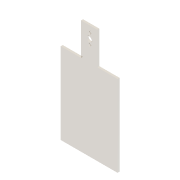
# Autodesk Inventor part: Ball Release
Saved by Autodesk Inventor 2015 SP1 (Build 190203100, 203)
## iProperties
Created: 2014-09-15
Part Number: Ball Release
Document SubType Name: Modeling
Designer: Family Room
Density: 1 g/cm^3
Material: Generic
Appearance: Polycarbonate - Smoked
Author: Family Room
Autodesk Inventor part; units mm, degrees
ref_plane "YZ Plane" through (0, 0, 0) normal (1, 0, 0) x (0, 1, 0)
ref_plane "XZ Plane" through (0, 0, 0) normal (0, 1, 0) x (-1, 0, 0)
ref_plane "XY Plane" through (0, 0, 0) normal (0, 0, 1) x (1, 0, 0)
sketch "Sketch1" plane through (0, 0, 0) normal (0, 0, 1) x (1, 0, 0)
  line L0 (0, 0) -> (88.9, 0)
  line L1 (88.9, 0) -> (88.9, 76.2)
  line L2 (0, 76.2) -> (0, 0)
  line L3 (57.15, 76.2) -> (57.15, 127)
  line L4 (57.15, 127) -> (31.75, 127)
  line L5 (31.75, 127) -> (31.75, 76.2)
  circle A0 centre (44.45, 107.95) radius 4
  circle A1 centre (44.45, 115.95) radius 1.85
  circle A2 centre (44.45, 99.95) radius 1.85
  line L6 (88.9, 76.2) -> (57.15, 76.2)
  line L7 (31.75, 76.2) -> (0, 76.2)
  point P0 (-8, 0)
  point P1 (8, 0)
  dimension "d0" = 88.9
  dimension "d1" = 76.2
  dimension "d2" = 25.4
  dimension "d3" = 50.8
  dimension "d7" = 8
  dimension "d8" = 8
  dimension "d9" = 19.05
  dimension "d10" = 12.7
  dimension "d11" = 31.75
  constraints: 16 end point, 4 parallel, 3 centre point, 1 horizontal, 1 perpendicular
  measures "d0" distance of L2.start L1.end
  measures "d1" distance of L1.end L0.end
  measures "d2" distance of L4.end L3.end
  measures "d3" distance of L3.end L3.start
  measures "d7" distance of A0.centre A1.centre
  measures "d8" distance of A2.centre A0.centre
  measures "d9" distance from line of L4 A0.centre
  measures "d10" distance from line of L5 A0.centre
  measures "d11" distance between parallel lines of L2 L5
extrude "Extrusion1" add sketch "Sketch1" along normal blind 3.175
sketch "Sketch2" plane through (0, 0, 0) normal (0, -1, 0) x (1, 0, 0)
  line L0 (88.9, 3.175) -> (0, 3.175) projected
  line L1 (0, 0) -> (0, 3.175) projected
  line L2 (0, 0) -> (88.9, 0) projected
  line L3 (88.9, 0) -> (88.9, 3.175) projected
extrude "Extrusion2" add sketch "Sketch2" along normal blind 50.8
body "Solid1"
